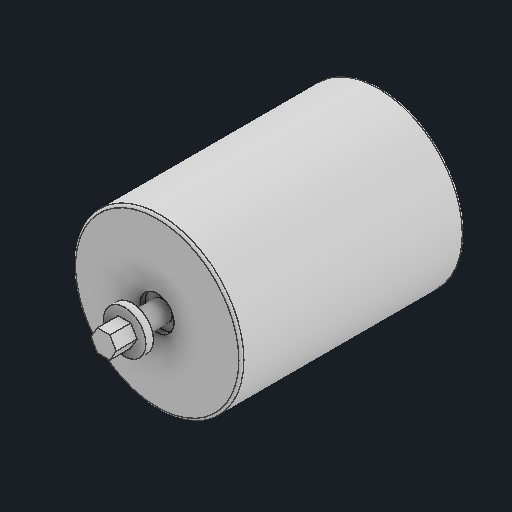
# Autodesk Inventor part: MY6812-12VDC-120W
Saved by Autodesk Inventor 2025.2 (Build 292293000, 293)
## iProperties
Created: 2025-10-04
Part Number: MY6812-12VDC-120W
Material: Generic
Document SubType Name: Modeling
Designer: valer
Density: 1 g/cm^3
Appearance: Default
Author: valer
Autodesk Inventor part; units mm, degrees
ref_plane "YZ Plane" through (0, 0, 0) normal (1, 0, 0) x (0, 1, 0)
ref_plane "XZ Plane" through (0, 0, 0) normal (0, 1, 0) x (-1, 0, 0)
sketch "Sketch1" plane through (0, 0, 0) normal (0, 0, 1) x (1, 0, 0)
  circle A0 centre (0, 0) radius 33.5
  dimension "d0" = 67
  constraints: 1 centre point, 1 coincident
  measures "d0" diameter of A0
extrude "Extrusion1" add sketch "Sketch1" along normal blind 89
sketch "Sketch2" plane through (0, 0, 0) normal (0, 0, -1) x (-1, 0, 0)
  circle A0 centre (0, 0) radius 14.75
  dimension "d3" = 29.5
  constraints: 1 centre point, 1 coincident
  measures "d3" diameter of A0
extrude "Extrusion2" add sketch "Sketch2" along normal blind 11
fillet "Fillet1" radius 1 3 edges at (14.75, 0, -11) (-33.5, 0, 0) (-33.5, 0, 89)
sketch "Sketch3" plane through (0, 0, 89) normal (0, 0, 1) x (1, 0, 0)
  circle A0 centre (0, 0) radius 33.5 projected
  circle A1 centre (0, 0) radius 6.75
  dimension "d7" = 13.5
  constraints: 1 centre point, 1 coincident
  measures "d7" diameter of A1
extrude "Extrusion3" cut sketch "Sketch3" against normal blind 2 contours A1
sketch "Sketch4" plane through (0, 0, 87) normal (0, 0, 1) x (1, 0, 0)
  circle A0 centre (0, 0) radius 4
  dimension "d10" = 8
  constraints: 1 centre point, 1 coincident
  measures "d10" diameter of A0
ref_plane "Work Plane1" through (0, 0, 99) normal (0, 0, 1) x (1, 0, 0)
extrude "Extrusion4" add sketch "Sketch4" along normal up to surface (12 mm away)
sketch "Sketch5" plane through (0, 0, 99) normal (0, 0, 1) x (1, 0, 0)
  circle A0 centre (0, 0) radius 32.5 construction
  circle A1 centre (0, 0) radius 8.5
  dimension "d14" = 17
  constraints: 1 centre point, 1 coincident
  measures "d14" diameter of A1
extrude "Extrusion5" add sketch "Sketch5" along normal blind 3
sketch "Sketch6" plane through (0, 0, 102) normal (0, 0, 1) x (1, 0, 0)
  circle A0 centre (0, 0) radius 8.5 projected
  line L0 (-2.5, 4.3301) -> (2.5, 4.3301)
  line L1 (2.5, 4.3301) -> (5, 0)
  line L2 (5, 0) -> (2.5, -4.3301)
  line L3 (2.5, -4.3301) -> (-2.5, -4.3301)
  line L4 (-2.5, -4.3301) -> (-5, 0)
  line L5 (-5, 0) -> (-2.5, 4.3301)
  line L6 (-46.9, 0) -> (46.9, 0) construction
  dimension "d17" = 10
  constraints: 12 end point, 1 coincident, 1 point on line, 13 other
  measures "d17" distance of L1.end L4.end
extrude "Extrusion6" add sketch "Sketch6" along normal blind 8.33 contours L0 L1 L2 L3 L4 L5
body "Solid1"
